Autodesk Fusion 360 part; units mm, degrees
note: some values were not read from the file. Chosen so that the rebuilt part matches the saved one: which face or edge a step refers to.
(part 2 of 2)
sketch "Sketch4 (10)" plane through (14, 0, 0) normal (1, 0, 0) x (0, 0, -1) in component "top v5 (2)"
  line L0 (21, 1) -> (21, 9)
  line L1 (21, 9) -> (20, 9)
  line L2 (20, 9) -> (20, 1)
  line L3 (20, 1) -> (21, 1)
  line L4 (21, 2.5) -> (25, 2.5) construction
  circle A0 centre (25, 2.5) radius 1.5
  line L5 (0, 0) -> (20, 0)
  circle A1 centre (25, 2.5) radius 1
  line L6 (21, 4) -> (25, 4)
  line L7 (21, 1) -> (25, 1)
  dimension "d22_9" = 3
  dimension "d24_7" = 4
  dimension "d26_8" = 2
  dimension "d27_9" = 1.5
  constraint coincident L0 L4.start
  constraint perpendicular L0 L4
  constraint coincident L4.end A0.centre
  constraint concentric A0 A1
  constraint coincident L0 L6.start
  constraint perpendicular L0 L6
  constraint tangent A0 L6
  constraint horizontal L7
  constraint tangent A0 L7
  constraint coincident A0 L6.end
  constraint coincident L0.start L3.end
  constraint coincident A0 L7.end
  measures "d22_9" diameter of A0
  measures "d24_7" distance of L4.start L4.end
  measures "d26_8" diameter of A1
  measures "d27_9" distance of L3 L4
extrude "Extrude3'''''''''" add sketch "Sketch4 (10)" against normal blind 3 contours L0 A0 L6 L7 | A0 bodies 10 in component "top v5 (2)"
sketch "Sketch5 (10)" plane through (1, 0, 0) normal (-1, 0, 0) x (0, 0, 1) in component "top v5 (2)"
  line L0 (-21, 9) -> (-21, 1)
  line L1 (-21, 1) -> (-20, 1)
  line L2 (-20, 1) -> (-20, 9)
  line L3 (-20, 9) -> (-21, 9)
  circle A0 centre (-25, 2.5) radius 1.5
  circle A1 centre (-25, 2.5) radius 1
  line L4 (-25, 4) -> (-21, 4)
  line L5 (-21, 1) -> (-25, 1)
  line L6 (-21, 2.5) -> (-25, 2.5) construction
  point P0 (-25, 2.5)
  dimension "d31_9" = 3
  dimension "d32_9" = 2
  dimension "d33_3" = 3
  dimension "d34_3" = 4
  constraint concentric A0 A1
  constraint coincident L0 L4.end
  constraint perpendicular L0 L4
  constraint coincident L0.end L1.start
  constraint perpendicular L0 L5
  constraint coincident A0 L5.end
  constraint tangent A0 L4
  constraint coincident A0 L4.start
  constraint coincident L0 L6.start
  constraint coincident P0 A0.centre
  constraint coincident L6 P0
  measures "d31_9" diameter of A0
  measures "d32_9" diameter of A1
  measures "d33_3" distance of L4 L5
  measures "d34_3" distance of L6.start P0
extrude "Extrude4'''''" add sketch "Sketch5 (10)" against normal blind 3 contours L0 A0 L4 L5 | A0 bodies 10 in component "top v5 (2)"
sketch "Sketch6 (8)" plane through (0, 0, 0) normal (0, -1, 0) x (1, 0, 0) in component "top v5 (2)"
  line L0 (0, 0) -> (0, -20)
  line L1 (0, -20) -> (15, -20)
  line L2 (15, -20) -> (15, 0)
  line L3 (15, 0) -> (0, 0)
sketch "Sketch7 (6)" plane through (0, 0, -21) normal (0, 0, -1) x (-1, 0, 0) in component "top v5 (2)"
  line L0 (-4, 4) -> (-1, 4)
  line L1 (-1, 4) -> (-1, 9)
  line L2 (-1, 9) -> (-14, 9)
  line L3 (-14, 9) -> (-14, 4)
  line L4 (-14, 4) -> (-11, 4)
  line L5 (-11, 4) -> (-11, 1)
  line L6 (-11, 1) -> (-4, 1)
  line L7 (-4, 1) -> (-4, 4)
sketch "Sketch8 (6)" plane through (0, 0, -21) normal (0, 0, -1) x (-1, 0, 0) in component "top v5 (2)"
sketch "Sketch9 (6)" plane through (0, 0, 0) normal (0, 0, 1) x (1, 0, 0) in component "top v5 (2)"
  line L0 (0, 3) -> (0, 0)
  line L1 (0, 0) -> (15, 0)
  line L2 (15, 0) -> (15, 3)
  line L3 (15, 3) -> (0, 3)
  circle A0 centre (2.5, 5.5) radius 1.5
  line L4 (0, 10) -> (0, 3)
  line L5 (7.5, 3) -> (7.5, 9.6608) construction
  circle A1 centre (12.5, 5.5) radius 1.5
  dimension "d41_2" = 3
  dimension "d42_3" = 2.5
  dimension "d43_3" = 2.5
  constraint midpoint L3 L5.start
  constraint perpendicular L3 L5
  constraint symmetric A0 L5 A1
  measures "d41_2" diameter of A0
  measures "d42_3" distance of L3 A0.centre
  measures "d43_3" distance of A0.centre L4
extrude "Extrude5''" cut sketch "Sketch9 (6)" against normal blind 15 contours A0 | A1 bodies 10 in component "top v5 (2)"
sketch "Sketch10 (5)" plane through (0, 0, 0) normal (0, -1, 0) x (1, 0, 0) in component "top v5 (2)"
sketch "Sketch11 (5)" plane through (0, 0, 0) normal (0, -1, 0) x (1, 0, 0) in component "top v5 (2)"
sketch "Sketch12 (5)" plane through (0, 0, 0) normal (0, -1, 0) x (1, 0, 0) in component "top v5 (2)"
  line L0 (0, 0) -> (0, -20)
  line L1 (0, -20) -> (15, -20)
  line L2 (15, -20) -> (15, 0)
  line L3 (15, 0) -> (0, 0)
  spline S0 degree 5 poles (0, -2) (0.5838, -1.6896) (1.7517, -1.1357) (3.5045, -0.5055) (5.8468, -0.0305) (8.8064, 0.0199) (11.2274, -0.4094) (13.0916, -1.0608) (14.3597, -1.6595) (15, -2) knots 0 0 0 0 0 0 0.2 0.4 0.6 0.8 1 1 1 1 1 1
  line L4 (13.4574, -1.1798) -> (16.5426, -2.8202)
  line L5 (15, -20) -> (15, 0)
  line L6 (-1.4063, -2.7478) -> (1.4063, -1.2522)
  line L7 (0, 0) -> (0, -20)
  line L8 (0, -2) -> (0, 0)
  line L9 (15, 0) -> (15, -2)
  dimension "d46_3" = 62
  dimension "d47_3" = 62
  dimension "d53_2" = 2
  dimension "d54_2" = 2
  constraint coincident L0 S0.start
  constraint coincident L2 S0.end
  constraint midpoint S0.end L4
  constraint midpoint S0.start L6
  constraint coincident L0.start L3.end
  constraint coincident L2.end L3.start
  measures "d46_3" angle of L4 L5
  measures "d47_3" angle of L6 L7
  measures "d53_2" distance of L0.start S0.start
  measures "d54_2" distance of S0.end L2.end
extrude "Extrude6''" cut sketch "Sketch12 (5)" against normal through all contours L0 L2 L3 S0 L5 L7 L8 L9 bodies 10 in component "top v5 (2)"
sketch "Sketch1 (11)" plane through (0, 0, 0) normal (0, 1, 0) x (1, 0, 0) in component "middle v4 (2)"
  line L0 (7.5, -10) -> (-7.5, -10)
  line L1 (-7.5, -10) -> (-7.5, 10)
  line L2 (-7.5, 10) -> (7.5, 10)
  line L3 (7.5, 10) -> (7.5, -10)
  line L4 (7.5, -10) -> (-7.5, 10) construction
  line L5 (-7.5, -10) -> (7.5, 10) construction
  dimension "d4_10" = 15
  dimension "d5_14" = 20
  constraint horizontal L0
  constraint perpendicular L0 L1
  constraint parallel L0 L2
  constraint parallel L1 L3
  constraint coincident L4 origin
  constraint coincident L5 origin
  measures "d4_10" distance of L1.end L2.end
  measures "d5_14" distance of L0.start L2.end
extrude "Extrude1''''''''''" add sketch "Sketch1 (11)" along normal blind 10 separate body makes body 11 in component "middle v4 (2)"
sketch "Sketch2 (11)" plane through (0, 0, -10) normal (0, 0, -1) x (-1, 0, 0) in component "middle v4 (2)"
  line L0 (-7.5, 0) -> (7.5, 0)
  line L1 (7.5, 0) -> (7.5, 10)
  line L2 (7.5, 10) -> (-7.5, 10)
  line L3 (-7.5, 10) -> (-7.5, 0)
sketch "Sketch3 (11)" plane through (0, 0, -10) normal (0, 0, -1) x (-1, 0, 0) in component "middle v4 (2)"
  line L0 (-6.5, 9) -> (6.5, 9)
  line L1 (6.5, 9) -> (6.5, 1)
  line L2 (6.5, 1) -> (-6.5, 1)
  line L3 (-6.5, 1) -> (-6.5, 9)
  line L4 (7.5, 10) -> (-7.5, 10)
  line L5 (-7.5, 10) -> (-7.5, 0)
  dimension "d11_5" = 8
  dimension "d12_8" = 13
  dimension "d13_8" = 1
  dimension "d14_4" = 1
  constraint horizontal L0
  constraint vertical L1
  constraint horizontal L2
  constraint vertical L3
  measures "d11_5" distance of L0.end L1.end
  measures "d12_8" distance of L0.start L0.end
  measures "d13_8" distance of L0 L4
  measures "d14_4" distance of L3 L5
extrude "Extrude2''''''''''" add sketch "Sketch3 (11)" along normal blind 1 bodies 11 in component "middle v4 (2)"
sketch "Sketch4 (11)" plane through (0, 0, -11) normal (0, 0, -1) x (-1, 0, 0) in component "middle v4 (2)"
  line L0 (-6.5, 1) -> (6.5, 1)
  line L1 (6.5, 1) -> (6.5, 9)
  line L2 (6.5, 9) -> (-6.5, 9)
  line L3 (-6.5, 9) -> (-6.5, 1)
ref_plane "WorkPlane1" through (0, 5, -10.5) normal (1, 0, 0) x (0, -1, 0) in component "middle v4 (2)"
sketch "Sketch5 (11)" plane through (0, 5, -10.5) normal (1, 0, 0) x (0, 0, -1) in component "middle v4 (2)"
sketch "Sketch6 (9)" plane through (0, 0, -11) normal (0, 0, -1) x (-1, 0, 0) in component "middle v4 (2)"
sketch "Sketch7 (7)" plane through (0, 0, -11) normal (0, 0, -1) x (-1, 0, 0) in component "middle v4 (2)"
sketch "Sketch8 (7)" plane through (0, 0, -11) normal (0, 0, -1) x (1, 0, 0) in component "middle v4 (2)"
sketch "Sketch9 (7)" plane through (0, 5, -10.5) normal (1, 0, 0) x (0, 0, -1) in component "middle v4 (2)"
sketch "Sketch10 (6)" plane through (0, 5, -10.5) normal (1, 0, 0) x (0, 0, -1) in component "middle v4 (2)"
sketch "Sketch11 (6)" plane through (0, 5, -10.5) normal (1, 0, 0) x (0, 0, -1) in component "middle v4 (2)"
  line L0 (0, 0) -> (0.5, 0) construction
  line L1 (0.5, 0) -> (0.5, -4) construction
  circle A0 centre (3, -2.5) radius 1
  circle A1 centre (3, -2.5) radius 1.5
  line L2 (0.5, -2.5) -> (3, -2.5) construction
  line L3 (0.5, -4) -> (3, -4)
  line L4 (0.5, -1) -> (3, -1)
  line L5 (0.5, -1) -> (0.5, -4)
  dimension "d18_9" = 0.5
  dimension "d19_8" = 4
  dimension "d22_10" = 3
  dimension "d23_5" = 2
  dimension "d25_10" = 2.5
  constraint coincident L0.start origin
  constraint horizontal L0
  constraint perpendicular L0 L1
  constraint concentric A0 A1
  constraint coincident L1 L2.start
  constraint perpendicular L1 L2
  constraint coincident A0.centre A1.centre
  constraint perpendicular L1 L3
  constraint tangent A1 L3
  constraint coincident A1 L3.end
  constraint coincident L1 L4.start
  constraint perpendicular L1 L4
  constraint tangent A1 L4
  constraint coincident A1 L4.end
  measures "d18_9" distance of L0.start L0.end
  measures "d19_8" distance of L0.end L1.end
  measures "d22_10" diameter of A1
  measures "d23_5" diameter of A0
  measures "d25_10" distance of L2.start A0.centre
sketch "Sketch12 (6)" plane through (0, 5, -10.5) normal (1, 0, 0) x (0, 0, -1) in component "middle v4 (2)"
extrude "Extrude3''''''''''" add sketch "Sketch11 (6)" along normal blind 3.5 and the other way blind 3.5 bodies 11 in component "middle v4 (2)"
ref_plane "WorkPlane2" through (0, 5, 0) normal (0, 0, 1) x (1, 0, 0) in component "middle v4 (2)"
mirror "Mirror1''''" about plane through (0, 5, 0) normal (0, 0, 1) of "Extrude2''''''''''", "Extrude3''''''''''" in component "middle v4 (2)"
sketch "Sketch1 (12)" plane through (0, 0, 0) normal (0, 1, 0) x (1, 0, 0) in component "end v6 (2)"
  line L0 (7.5, -15) -> (-7.5, -15)
  line L1 (-7.5, -15) -> (-7.5, 15)
  line L2 (-7.5, 15) -> (7.5, 15)
  line L3 (7.5, 15) -> (7.5, -15)
  line L4 (7.5, -15) -> (-7.5, 15) construction
  line L5 (-7.5, -15) -> (7.5, 15) construction
  dimension "d4_11" = 30
  dimension "d5_15" = 15
  constraint horizontal L0
  constraint perpendicular L0 L1
  constraint parallel L0 L2
  constraint parallel L1 L3
  constraint coincident L4 origin
  constraint coincident L5 origin
  measures "d4_11" distance of L0.start L2.end
  measures "d5_15" distance of L0.start L0.end
extrude "Extrude1'''''''''''" add sketch "Sketch1 (12)" along normal blind 10 separate body makes body 12 in component "end v6 (2)"
sketch "Sketch2 (12)" plane through (0, 0, -15) normal (0, 0, -1) x (-1, 0, 0) in component "end v6 (2)"
  line L0 (-7.5, 0) -> (7.5, 0)
  line L1 (7.5, 0) -> (7.5, 10)
  line L2 (7.5, 10) -> (-7.5, 10)
  line L3 (-7.5, 10) -> (-7.5, 0)
  line L4 (-6.5, 9) -> (6.5, 9)
  line L5 (6.5, 9) -> (6.5, 1)
  line L6 (6.5, 1) -> (-6.5, 1)
  line L7 (-6.5, 1) -> (-6.5, 9)
  dimension "d10_3" = 13
  dimension "d11_6" = 8
  dimension "d12_9" = 1
  dimension "d13_9" = 1
  constraint horizontal L4
  constraint vertical L5
  constraint horizontal L6
  constraint vertical L7
  measures "d10_3" distance of L4.start L4.end
  measures "d11_6" distance of L4.end L5.end
  measures "d12_9" distance of L2 L4
  measures "d13_9" distance of L3 L7
extrude "Extrude2'''''''''''" add sketch "Sketch2 (12)" along normal blind 1 contours L4 L5 L6 L7 bodies 12 in component "end v6 (2)"
ref_plane "WorkPlane1" through (0, 5, -15.5) normal (1, 0, 0) x (0, -1, 0) in component "end v6 (2)"
sketch "Sketch3 (12)" plane through (6.5, 0, 0) normal (1, 0, 0) x (0, 0, -1) in component "end v6 (2)"
  line L0 (15, 9) -> (15, 1)
  line L1 (15, 1) -> (16, 1)
  line L2 (16, 1) -> (16, 9)
  line L3 (16, 9) -> (15, 9)
  line L4 (16, 1) -> (18.5, 1)
  line L5 (16, 2.5) -> (18.5, 2.5) construction
  circle A0 centre (18.5, 2.5) radius 1.5
  circle A1 centre (18.5, 2.5) radius 1
  line L6 (16, 4) -> (18.5, 4)
  dimension "d20_11" = 2.5
  dimension "d21_2" = 3
  dimension "d22_11" = 2
  constraint coincident L1.end L2.start
  constraint perpendicular L2 L4
  constraint coincident L2 L5.start
  constraint perpendicular L2 L5
  constraint coincident L5.end A0.centre
  constraint concentric A0 A1
  constraint coincident L2 L6.start
  constraint perpendicular L2 L6
  constraint tangent L4 A0
  constraint tangent A0 L6
  constraint coincident A0 L6.end
  constraint coincident L4.end A0
  measures "d20_11" distance of L5.start L5.end
  measures "d21_2" diameter of A0
  measures "d22_11" diameter of A1
extrude "Extrude3'''''''''''" add sketch "Sketch3 (12)" against normal blind 3 contours L2 L4 A0 L6 | A0 bodies 12 in component "end v6 (2)"
mirror "Mirror1'''''" about plane through (0, 5, -15.5) normal (1, 0, 0) of "Extrude2'''''''''''", "Extrude3'''''''''''" in component "end v6 (2)"
ref_plane "WorkPlane2" through (0, 5, 0) normal (0, 0, 1) x (1, 0, 0) in component "end v6 (2)"
mirror "Mirror2''" about plane through (0, 5, 0) normal (0, 0, 1) of 13 faces at (3.5, 2.5, -16.5) (4.5, 3.4925, -19.6247) (5.5, 4, -16.8333) (-4.5, 3.5474, -19.5738) (-6.5, 2.5, -16.1667) (-5.5, 4, -16.8333) (1.1667, 7.3333, -16) (6.5, 2.5, -16.1667) (2.1667, 9, -15.3333) (5.5, 1, -16.5) (-3.5, 2.5, -16.5) (5.5, 2.4004, -19.495) (-5.5, 2.4004, -19.495) on bodies 12 in component "end v6 (2)"
sketch "Sketch4 (12)" plane through (0, 0, 15) normal (0, 0, 1) x (1, 0, 0) in component "end v6 (2)"
  line L0 (6.5, 9) -> (6.5, 1)
  line L1 (6.5, 1) -> (-6.5, 1)
  line L2 (-6.5, 1) -> (-6.5, 9)
  line L3 (-6.5, 9) -> (6.5, 9)
  line L4 (-7.5, 0) -> (7.5, 0)
  line L5 (7.5, 0) -> (7.5, 10)
  line L6 (7.5, 10) -> (-7.5, 10)
  line L7 (-7.5, 10) -> (-7.5, 0)
sketch "Sketch5 (12)" plane through (6.5, 0, 0) normal (1, 0, 0) x (0, 0, -1) in component "end v6 (2)"
  circle A0 centre (-18.5, 2.5) radius 1
  line L0 (-16, 9) -> (-16, 4)
  line L1 (-16, 4) -> (-18.5, 4)
  arc A1 (-18.5, 4) -> (-18.5, 1) centre (-18.5, 2.5) ccw
  line L2 (-18.5, 1) -> (-15, 1)
  line L3 (-15, 1) -> (-15, 9)
  line L4 (-15, 9) -> (-16, 9)
sketch "Sketch6 (10)" plane through (0, 0, 16) normal (0, 0, 1) x (1, 0, 0) in component "end v6 (2)"
  line L0 (-3.5, 4) -> (-3.5, 1)
  line L1 (-3.5, 1) -> (3.5, 1)
  line L2 (3.5, 1) -> (3.5, 4)
  line L3 (3.5, 4) -> (6.5, 4)
  line L4 (6.5, 4) -> (6.5, 9)
  line L5 (6.5, 9) -> (-6.5, 9)
  line L6 (-6.5, 9) -> (-6.5, 4)
  line L7 (-6.5, 4) -> (-3.5, 4)
fillet "Fillet1''''" radius 3 1 edges at (0, 0, 15) on bodies 12 in component "end v6 (2)"
sketch "Sketch1 (13)" plane through (0, 0, 0) normal (1, 0, 0) x (0, 0, -1) in component "turner v14 (2)"
  line L0 (10, -10) -> (-10, -10)
  line L1 (-10, -10) -> (-10, 10)
  line L2 (-10, 10) -> (10, 10)
  line L3 (10, 10) -> (10, -10)
  line L4 (10, -10) -> (-10, 10) construction
  line L5 (-10, -10) -> (10, 10) construction
  dimension "d4_12" = 20
  dimension "d5_16" = 20
  constraint horizontal L0
  constraint perpendicular L0 L1
  constraint parallel L0 L2
  constraint parallel L1 L3
  constraint coincident L4 origin
  constraint coincident L5 origin
  measures "d4_12" distance of L0.start L2.end
  measures "d5_16" distance of L0.start L0.end
extrude "Extrude1''''''''''''" add sketch "Sketch1 (13)" along normal blind 20 separate body makes body 13 in component "turner v14 (2)"
sketch "Sketch2 (13)" plane through (0, 0, -10) normal (0, 0, -1) x (-1, 0, 0) in component "turner v14 (2)"
  line L0 (0, -10) -> (0, 10)
  line L1 (0, 10) -> (-20, 10)
  line L2 (-20, 10) -> (-20, -10)
  line L3 (-20, -10) -> (0, -10)
  line L4 (-10, 10) -> (-3.5, 10)
  line L5 (-3.5, 10) -> (-3.5, 3.5)
  line L6 (-10, 10) -> (-10, 4.4853) construction
  line L7 (-10, 10) -> (-16.5, 10)
  line L8 (-16.5, 10) -> (-16.5, 3.5)
  arc A0 (-16.5, 3.5) -> (-3.5, 3.5) centre (-10, 3.5) ccw
  dimension "d12_10" = 6.5
  dimension "d13_10" = 6.5
  constraint midpoint L1 L4.start
  constraint parallel L1 L4
  constraint perpendicular L4 L5
  constraint perpendicular L1 L6
  constraint symmetric L4.start L6 L7.start
  constraint symmetric L4.end L6 L7.end
  constraint symmetric L5.end L6 L8.end
  constraint tangent L5 A0
  measures "d12_10" distance of L4.start L4.end
  measures "d13_10" distance of L4.end L5.end
extrude "Extrude2''''''''''''" cut sketch "Sketch2 (13)" against normal blind 10 contours L1 L4 L5 L7 L8 A0 bodies 13 in component "turner v14 (2)"
sketch "Sketch3 (13)" plane through (3.5, 0, 0) normal (1, 0, 0) x (0, 0, -1) in component "turner v14 (2)"
  line L0 (10, 3.5) -> (10, 10)
  line L1 (10, 10) -> (0, 10)
  line L2 (0, 10) -> (0, 3.5)
  line L3 (0, 3.5) -> (10, 3.5)
  line L4 (5, 3.5) -> (5, 7.5) construction
  circle A0 centre (5, 7.5) radius 1
  dimension "d20_12" = 4
  dimension "d22_12" = 5
  dimension "d23_6" = 2
  constraint coincident L3 L4.start
  constraint perpendicular L3 L4
  constraint coincident L4.end A0.centre
  measures "d20_12" distance of L4.start L4.end
  measures "d22_12" distance of L0 L4
  measures "d23_6" diameter of A0
extrude "Extrude3''''''''''''" add sketch "Sketch3 (13)" along normal up to surface (13 mm away) contours A0 bodies 13 in component "turner v14 (2)"
sketch "Sketch4 (13)" plane through (0, 0, 10) normal (0, 0, 1) x (1, 0, 0) in component "turner v14 (2)"
  line L0 (0, 10) -> (0, -10)
  line L1 (0, -10) -> (20, -10)
  line L2 (20, -10) -> (20, 10)
  line L3 (20, 10) -> (0, 10)
sketch "Sketch5 (13)" plane through (0, 0, 10) normal (0, 0, 1) x (1, 0, 0) in component "turner v14 (2)"
  circle A0 centre (10, 0) radius 1.5
  line L0 (20, 10) -> (0, 10)
  line L1 (20, -10) -> (20, 10)
  dimension "d28_11" = 3
  dimension "d29_15" = 10
  dimension "d30_12" = 10
  measures "d28_11" diameter of A0
  measures "d29_15" distance of A0.centre L0
  measures "d30_12" distance of A0.centre L1
extrude "Extrude4''''''" add sketch "Sketch5 (13)" along normal blind 3 bodies 13 in component "turner v14 (2)"
fillet "Fillet1'''''" radius 7 1 edges at (10, -10, -10) on bodies 13 in component "turner v14 (2)"
fillet "Fillet2''" radius 7 3 edges at (20, -10, 3.5) (20, -7.9497, -7.9497) (20, 3.5, -10) on bodies 13 in component "turner v14 (2)"
fillet "Fillet3''" radius 7 3 edges at (0, 3.5, -10) (0, -7.9497, -7.9497) (0, -10, 3.5) on bodies 13 in component "turner v14 (2)"
component "base v7" placed x (1, 0, 0) y (0, 1, 0) z (0, 0, 1) at (0, 0, 0)
component "test v8" placed x (1, 0, 0) y (0, 1, 0) z (0, 0, 1) at (0, 0, 60)
component "test v8 (1)" placed x (1, 0, 0) y (0, 1, 0) z (0, 0, 1) at (50, 0, 0)
component "test v8 (2)" placed x (-0.816035, -0.071394, 0.573576) y (-0.087156, 0.996195, 0) z (-0.571394, -0.04999, -0.819152) at (50, 0, 0)
component "top v5" placed x (1, 0, 0) y (0, 0.258819, -0.965926) z (0, 0.965926, 0.258819) at (12.5, 145.8984, -86.2615) in component "test v8"
component "middle v4" placed x (-1, 0, 0) y (0, 0.087156, -0.996195) z (0, -0.996195, -0.087156) at (20, 108.7307, -93.8329) in component "test v8"
component "end v6" placed x (-1, 0, 0) y (0, 0, -1) z (0, -1, 0) at (20, 77, -95) in component "test v8"
component "turner v14" placed x (1, 0, 0) y (0, 1, 0) z (0, 0, 1) at (10, 51, -92.5) in component "test v8"
component "top v5 (1)" placed x (1, 0, 0) y (0, 0.258819, -0.965926) z (0, 0.965926, 0.258819) at (-77.5, 145.8984, -26.2615) in component "test v8 (1)"
component "middle v4 (1)" placed x (-1, 0, 0) y (0, 0.087156, -0.996195) z (0, -0.996195, -0.087156) at (-70, 108.7307, -33.8329) in component "test v8 (1)"
component "end v6 (1)" placed x (-1, 0, 0) y (0, 0, -1) z (0, -1, 0) at (-70, 77, -35) in component "test v8 (1)"
component "turner v14 (1)" placed x (1, 0, 0) y (0, 1, 0) z (0, 0, 1) at (-80, 51, -32.5) in component "test v8 (1)"
component "top v5 (2)" placed x (0.816035, 0.087156, 0.571394) y (0.535554, 0.257834, -0.804179) z (-0.217414, 0.96225, 0.163725) at (39.3282, 149.0473, -4.5215) in component "test v8 (2)"
component "middle v4 (2)" placed x (-0.816035, -0.087156, -0.571394) y (0.565171, 0.086824, -0.820392) z (0.121113, -0.992404, -0.021594) at (52.4448, 112.6748, -4.5801) in component "test v8 (2)"
component "end v6 (2)" placed x (-0.816035, -0.087156, -0.571394) y (0.573576, 0, -0.819152) z (0.071394, -0.996195, 0.04999) at (55.3796, 81.0648, -3.9499) in component "test v8 (2)"
component "turner v14 (2)" placed x (0.816035, 0.087156, 0.571394) y (-0.071394, 0.996195, -0.04999) z (-0.573576, 0, 0.819152) at (47.6415, 54.2922, -6.3162) in component "test v8 (2)"
equation "base_sq = 95 mm"
equation "base_circ = 60 mm"
equation "d3_1 = base_circ"
equation "base_circ_sq_dist = 30 mm"
equation "d5_1 = base_circ_sq_dist"
equation "d6_1 = base_sq"
equation "d7_1 = base_sq"
equation "sq1_sq2_dist = 7 mm"
equation "d9_1 = sq1_sq2_dist"
equation "up_sq = 80 mm"
equation "up_dw_sq_dist = 25 mm"
equation "d12_1 = up_dw_sq_dist"
equation "d13_1 = up_sq"
equation "d14_1 = up_sq"
equation "cut_sq_h = 22 mm"
equation "cut_sq_width = 22 mm"
equation "d17 = cut_sq_h"
equation "d18 = cut_sq_width"
equation "middle_width = ( up_sq - cut_sq_width ) / 2"
equation "d20 = middle_width"
equation "cut_dist = 25 mm"
equation "d22 = -cut_dist"
equation "d23 = cut_sq_h"
equation "d24 = cut_sq_width"
equation "d25 = middle_width"
equation "screw_hole = 3 mm"
equation "screq_hole_ext = 3 mm"
equation "d29 = screw_hole"
equation "d30 = cut_sq_h / 2"
equation "d31 = cut_sq_width / 2"
equation "d32 = -screq_hole_ext"
equation "d34 = -cut_dist"
equation "d35 = cut_sq_h"
equation "d36 = rotate_sq_width"
equation "d37 = cut_sq_h"
equation "d38 = rotate_sq_width"
equation "rotate_sq_width = 25 mm"
equation "two_rotate_dist = 15 mm"
equation "rotate_mid_width = ( up_sq - 2 * rotate_sq_width - two_rotate_dist ) / 2"
equation "d42 = rotate_mid_width"
equation "d43 = rotate_mid_width"
equation "d45 = screw_hole"
equation "d46 = cut_sq_h / 2"
equation "d47 = rotate_sq_width / 2"
equation "d48 = screw_hole"
equation "d49 = rotate_sq_width / 2"
equation "d50 = cut_sq_h / 2"
equation "d51 = -screq_hole_ext"
equation "hight = 10 mm"
equation "width = 20 mm"
equation "ext = 15 mm"
equation "small_hight = 3 mm"
equation "d5_3 = width"
equation "d6_3 = hight"
equation "d7_3 = small_hight"
equation "d8_2 = ext"
equation "SND_SQ_DIST = 1 mm"
equation "snd_sq_width = 1 mm"
equation "snd_sq_hight = hight - 2 * SND_SQ_DIST"
equation "d16_1 = SND_SQ_DIST"
equation "d17_2 = ext - 2 * SND_SQ_DIST"
equation "d18_2 = snd_sq_hight"
equation "all_circ = 3 mm"
equation "d22_1 = all_circ"
equation "all_circ_dist = 4 mm"
equation "d24_1 = all_circ_dist"
equation "d26_2 = all_circ - 1 mm"
equation "d27_1 = all_circ / 2"
equation "all_circ_ext = 3 mm"
equation "d29_2 = -all_circ_ext"
equation "d31_1 = all_circ"
equation "d32_1 = all_circ - 1 mm"
equation "d33_1 = all_circ"
equation "d34_1 = all_circ_dist"
equation "d35_1 = -all_circ_ext"
equation "hole_cut = 15 mm"
equation "hole_cut_diam = 3 mm"
equation "cut_hole_dist_h = hole_cut_diam / 2 + 1 mm"
equation "cut_hole_dist_v = hole_cut_diam / 2 + 1 mm"
equation "d41 = hole_cut_diam"
equation "d42_1 = cut_hole_dist_v"
equation "d43_1 = cut_hole_dist_h"
equation "d44_1 = -hole_cut"
equation "d46_1 = spline_ang"
equation "d47_1 = spline_ang"
equation "spline_dist = 2 mm"
equation "spline_ang = 62 deg"
equation "d53 = spline_dist"
equation "d54 = spline_dist"
equation "width_1 = 15 mm"
equation "hight_1 = 20 mm"
equation "ext_1 = 10 mm"
equation "d4_2 = width_1"
equation "d5_4 = hight_1"
equation "d6_4 = ext_1"
equation "w = width_1 - 2 mm"
equation "h = ext_1 - 2 mm"
equation "exsmall_ext = 1 mm"
equation "d11_1 = h"
equation "d12_2 = w"
equation "d13_2 = ( ext_1 - h ) / 2"
equation "d14_2 = ( width_1 - w ) / 2"
equation "d15_1 = exsmall_ext"
equation "upper_hole_plane = ( w - 7 mm ) / 2"
equation "d19_2 = h / 2"
equation "all_circ_1 = 3 mm"
equation "all_circ_small = all_circ_1 - 1 mm"
equation "d22_2 = all_circ_1"
equation "d23_1 = all_circ_small"
equation "all_circ_dist_1 = 2.5 mm"
equation "d25_2 = all_circ_dist_1"
equation "all_circ_ext_1 = 3.5 mm"
equation "d27_2 = all_circ_ext_1"
equation "d29_3 = all_circ_ext_1"
equation "hight_2 = 30 mm"
equation "width_2 = 15 mm"
equation "ext_2 = 10 mm"
equation "d4_3 = hight_2"
equation "d5_5 = width_2"
equation "d6_5 = ext_2"
equation "h_1 = ext_2 - 2 mm"
equation "w_1 = width_2 - 2 mm"
equation "d10_1 = w_1"
equation "d11_2 = h_1"
equation "d12_3 = ( ext_2 - h_1 ) / 2"
equation "d13_3 = ( width_2 - w_1 ) / 2"
equation "small_ext = 1 mm"
equation "d15_2 = small_ext"
equation "all_circ_dist_2 = 2.5 mm"
equation "alll_circ = 3 mm"
equation "small_all_circ = alll_circ - 1 mm"
equation "d20_3 = all_circ_dist_2"
equation "d21 = alll_circ"
equation "d22_3 = small_all_circ"
equation "hole_big_ext = ( w_1 - 7 mm ) / 2"
equation "d24_2 = -hole_big_ext"
equation "end_fill = 3 mm"
equation "d32_3 = end_fill"
equation "sq_hight = 20 mm"
equation "sq_width = 20 mm"
equation "sq_ext = 20 mm"
equation "d4_4 = sq_width"
equation "d5_6 = sq_hight"
equation "line_diam = 7 mm"
equation "d8_3 = sq_ext"
equation "bottom_fill = 7 mm"
equation "coil_hole_hight = 13 mm"
equation "d12_4 = coil_hole_hight / 2"
equation "d13_4 = coil_hole_hight / 2"
equation "ext_cut = 10 mm"
equation "d15_3 = -ext_cut"
equation "screq_hight = 4 mm"
equation "sqrew_diam = 2 mm"
equation "d20_4 = screq_hight"
equation "sc_dist_surf = screq_hight"
equation "d22_4 = screw_width"
equation "d23_2 = sqrew_diam"
equation "screw_hole_1 = 3 mm"
equation "screw_ext = 3 mm"
equation "d28_3 = screw_hole_1"
equation "d29_5 = sq_width / 2"
equation "d30_4 = sq_ext / 2"
equation "d31_4 = screw_ext"
equation "back_fill = 7 mm"
equation "side_fill = 7 mm"
equation "d36_2 = back_fill"
equation "d38_1 = side_fill"
equation "d40 = side_fill"
equation "screw_width = 5 mm"
equation "hight_3 = 10 mm"
equation "width_3 = 20 mm"
equation "ext_3 = 15 mm"
equation "small_hight_1 = 3 mm"
equation "d5_8 = width_3"
equation "d6_7 = hight_3"
equation "d7_7 = small_hight_1"
equation "d8_5 = ext_3"
equation "SND_SQ_DIST_1 = 1 mm"
equation "snd_sq_width_1 = 1 mm"
equation "snd_sq_hight_1 = hight_3 - 2 * SND_SQ_DIST_1"
equation "d16_5 = SND_SQ_DIST_1"
equation "d17_4 = ext_3 - 2 * SND_SQ_DIST_1"
equation "d18_5 = snd_sq_hight_1"
equation "all_circ_2 = 3 mm"
equation "d22_5 = all_circ_2"
equation "all_circ_dist_3 = 4 mm"
equation "d24_4 = all_circ_dist_3"
equation "d26_5 = all_circ_2 - 1 mm"
equation "d27_5 = all_circ_2 / 2"
equation "all_circ_ext_2 = 3 mm"
equation "d29_7 = -all_circ_ext_2"
equation "d31_5 = all_circ_2"
equation "d32_5 = all_circ_2 - 1 mm"
equation "d33_2 = all_circ_2"
equation "d34_2 = all_circ_dist_3"
equation "d35_3 = -all_circ_ext_2"
equation "hole_cut_1 = 15 mm"
equation "hole_cut_diam_1 = 3 mm"
equation "cut_hole_dist_h_1 = hole_cut_diam_1 / 2 + 1 mm"
equation "cut_hole_dist_v_1 = hole_cut_diam_1 / 2 + 1 mm"
equation "d41_1 = hole_cut_diam_1"
equation "d42_2 = cut_hole_dist_v_1"
equation "d43_2 = cut_hole_dist_h_1"
equation "d44_2 = -hole_cut_1"
equation "d46_2 = spline_ang"
equation "d47_2 = spline_ang"
equation "spline_dist_1 = 2 mm"
equation "spline_ang_1 = 62 deg"
equation "d53_1 = spline_dist_1"
equation "d54_1 = spline_dist_1"
equation "width_4 = 15 mm"
equation "hight_4 = 20 mm"
equation "ext_4 = 10 mm"
equation "d4_6 = width_4"
equation "d5_9 = hight_4"
equation "d6_8 = ext_4"
equation "w_2 = width_4 - 2 mm"
equation "h_2 = ext_4 - 2 mm"
equation "exsmall_ext_1 = 1 mm"
equation "d11_3 = h_2"
equation "d12_5 = w_2"
equation "d13_5 = ( ext_4 - h_2 ) / 2"
equation "d14_3 = ( width_4 - w_2 ) / 2"
equation "d15_4 = exsmall_ext_1"
equation "upper_hole_plane_1 = ( w_2 - 7 mm ) / 2"
equation "d19_5 = h_2 / 2"
equation "all_circ_3 = 3 mm"
equation "all_circ_small_1 = all_circ_3 - 1 mm"
equation "d22_6 = all_circ_3"
equation "d23_3 = all_circ_small_1"
equation "all_circ_dist_4 = 2.5 mm"
equation "d25_6 = all_circ_dist_4"
equation "all_circ_ext_3 = 3.5 mm"
equation "d27_6 = all_circ_ext_3"
equation "d29_8 = all_circ_ext_3"
equation "hight_5 = 30 mm"
equation "width_5 = 15 mm"
equation "ext_5 = 10 mm"
equation "d4_7 = hight_5"
equation "d5_10 = width_5"
equation "d6_9 = ext_5"
equation "h_3 = ext_5 - 2 mm"
equation "w_3 = width_5 - 2 mm"
equation "d10_2 = w_3"
equation "d11_4 = h_3"
equation "d12_6 = ( ext_5 - h_3 ) / 2"
equation "d13_6 = ( width_5 - w_3 ) / 2"
equation "small_ext_1 = 1 mm"
equation "d15_5 = small_ext_1"
equation "all_circ_dist_5 = 2.5 mm"
equation "alll_circ_1 = 3 mm"
equation "small_all_circ_1 = alll_circ_1 - 1 mm"
equation "d20_7 = all_circ_dist_5"
equation "d21_1 = alll_circ_1"
equation "d22_7 = small_all_circ_1"
equation "hole_big_ext_1 = ( w_3 - 7 mm ) / 2"
equation "d24_5 = -hole_big_ext_1"
equation "end_fill_1 = 3 mm"
equation "d32_7 = end_fill_1"
equation "sq_hight_1 = 20 mm"
equation "sq_width_1 = 20 mm"
equation "sq_ext_1 = 20 mm"
equation "d4_8 = sq_width_1"
equation "d5_11 = sq_hight_1"
equation "line_diam_1 = 7 mm"
equation "d8_6 = sq_ext_1"
equation "bottom_fill_1 = 7 mm"
equation "coil_hole_hight_1 = 13 mm"
equation "d12_7 = coil_hole_hight_1 / 2"
equation "d13_7 = coil_hole_hight_1 / 2"
equation "ext_cut_1 = 10 mm"
equation "d15_6 = -ext_cut_1"
equation "screq_hight_1 = 4 mm"
equation "sqrew_diam_1 = 2 mm"
equation "d20_8 = screq_hight_1"
equation "sc_dist_surf_1 = screq_hight_1"
equation "d22_8 = screw_width"
equation "d23_4 = sqrew_diam_1"
equation "screw_hole_2 = 3 mm"
equation "screw_ext_1 = 3 mm"
equation "d28_7 = screw_hole_2"
equation "d29_10 = sq_width_1 / 2"
equation "d30_8 = sq_ext_1 / 2"
equation "d31_8 = screw_ext_1"
equation "back_fill_1 = 7 mm"
equation "side_fill_1 = 7 mm"
equation "d36_4 = back_fill_1"
equation "d38_2 = side_fill_1"
equation "d40_1 = side_fill_1"
equation "screw_width_1 = 5 mm"
equation "hight_6 = 10 mm"
equation "width_6 = 20 mm"
equation "ext_6 = 15 mm"
equation "small_hight_2 = 3 mm"
equation "d5_13 = width_6"
equation "d6_11 = hight_6"
equation "d7_11 = small_hight_2"
equation "d8_8 = ext_6"
equation "SND_SQ_DIST_2 = 1 mm"
equation "snd_sq_width_2 = 1 mm"
equation "snd_sq_hight_2 = hight_6 - 2 * SND_SQ_DIST_2"
equation "d16_9 = SND_SQ_DIST_2"
equation "d17_6 = ext_6 - 2 * SND_SQ_DIST_2"
equation "d18_8 = snd_sq_hight_2"
equation "all_circ_4 = 3 mm"
equation "d22_9 = all_circ_4"
equation "all_circ_dist_6 = 4 mm"
equation "d24_7 = all_circ_dist_6"
equation "d26_8 = all_circ_4 - 1 mm"
equation "d27_9 = all_circ_4 / 2"
equation "all_circ_ext_4 = 3 mm"
equation "d29_12 = -all_circ_ext_4"
equation "d31_9 = all_circ_4"
equation "d32_9 = all_circ_4 - 1 mm"
equation "d33_3 = all_circ_4"
equation "d34_3 = all_circ_dist_6"
equation "d35_5 = -all_circ_ext_4"
equation "hole_cut_2 = 15 mm"
equation "hole_cut_diam_2 = 3 mm"
equation "cut_hole_dist_h_2 = hole_cut_diam_2 / 2 + 1 mm"
equation "cut_hole_dist_v_2 = hole_cut_diam_2 / 2 + 1 mm"
equation "d41_2 = hole_cut_diam_2"
equation "d42_3 = cut_hole_dist_v_2"
equation "d43_3 = cut_hole_dist_h_2"
equation "d44_3 = -hole_cut_2"
equation "d46_3 = spline_ang"
equation "d47_3 = spline_ang"
equation "spline_dist_2 = 2 mm"
equation "spline_ang_2 = 62 deg"
equation "d53_2 = spline_dist_2"
equation "d54_2 = spline_dist_2"
equation "width_7 = 15 mm"
equation "hight_7 = 20 mm"
equation "ext_7 = 10 mm"
equation "d4_10 = width_7"
equation "d5_14 = hight_7"
equation "d6_12 = ext_7"
equation "w_4 = width_7 - 2 mm"
equation "h_4 = ext_7 - 2 mm"
equation "exsmall_ext_2 = 1 mm"
equation "d11_5 = h_4"
equation "d12_8 = w_4"
equation "d13_8 = ( ext_7 - h_4 ) / 2"
equation "d14_4 = ( width_7 - w_4 ) / 2"
equation "d15_7 = exsmall_ext_2"
equation "upper_hole_plane_2 = ( w_4 - 7 mm ) / 2"
equation "d19_8 = h_4 / 2"
equation "all_circ_5 = 3 mm"
equation "all_circ_small_2 = all_circ_5 - 1 mm"
equation "d22_10 = all_circ_5"
equation "d23_5 = all_circ_small_2"
equation "all_circ_dist_7 = 2.5 mm"
equation "d25_10 = all_circ_dist_7"
equation "all_circ_ext_5 = 3.5 mm"
equation "d27_10 = all_circ_ext_5"
equation "d29_13 = all_circ_ext_5"
equation "hight_8 = 30 mm"
equation "width_8 = 15 mm"
equation "ext_8 = 10 mm"
equation "d4_11 = hight_8"
equation "d5_15 = width_8"
equation "d6_13 = ext_8"
equation "h_5 = ext_8 - 2 mm"
equation "w_5 = width_8 - 2 mm"
equation "d10_3 = w_5"
equation "d11_6 = h_5"
equation "d12_9 = ( ext_8 - h_5 ) / 2"
equation "d13_9 = ( width_8 - w_5 ) / 2"
equation "small_ext_2 = 1 mm"
equation "d15_8 = small_ext_2"
equation "all_circ_dist_8 = 2.5 mm"
equation "alll_circ_2 = 3 mm"
equation "small_all_circ_2 = alll_circ_2 - 1 mm"
equation "d20_11 = all_circ_dist_8"
equation "d21_2 = alll_circ_2"
equation "d22_11 = small_all_circ_2"
equation "hole_big_ext_2 = ( w_5 - 7 mm ) / 2"
equation "d24_8 = -hole_big_ext_2"
equation "end_fill_2 = 3 mm"
equation "d32_11 = end_fill_2"
equation "sq_hight_2 = 20 mm"
equation "sq_width_2 = 20 mm"
equation "sq_ext_2 = 20 mm"
equation "d4_12 = sq_width_2"
equation "d5_16 = sq_hight_2"
equation "line_diam_2 = 7 mm"
equation "d8_9 = sq_ext_2"
equation "bottom_fill_2 = 7 mm"
equation "coil_hole_hight_2 = 13 mm"
equation "d12_10 = coil_hole_hight_2 / 2"
equation "d13_10 = coil_hole_hight_2 / 2"
equation "ext_cut_2 = 10 mm"
equation "d15_9 = -ext_cut_2"
equation "screq_hight_2 = 4 mm"
equation "sqrew_diam_2 = 2 mm"
equation "d20_12 = screq_hight_2"
equation "sc_dist_surf_2 = screq_hight_2"
equation "d22_12 = screw_width"
equation "d23_6 = sqrew_diam_2"
equation "screw_hole_3 = 3 mm"
equation "screw_ext_2 = 3 mm"
equation "d28_11 = screw_hole_3"
equation "d29_15 = sq_width_2 / 2"
equation "d30_12 = sq_ext_2 / 2"
equation "d31_12 = screw_ext_2"
equation "back_fill_2 = 7 mm"
equation "side_fill_2 = 7 mm"
equation "d36_6 = back_fill_2"
equation "d38_3 = side_fill_2"
equation "d40_2 = side_fill_2"
equation "screw_width_2 = 5 mm"
